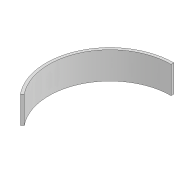
# Autodesk Inventor part: Ball_plate
Saved by Autodesk Inventor 2022 (Build 260153000, 153)
## iProperties
Created: 2022-08-08
Part Number: Ball_plate
Material: Generic
Document SubType Name: Modeling
Designer: dell
Density: 1 g/cm^3
Appearance: Default
Author: dell
Autodesk Inventor part; units mm, degrees
ref_plane "YZ Plane" through (0, 0, 0) normal (1, 0, 0) x (0, 1, 0)
ref_plane "XZ Plane" through (0, 0, 0) normal (0, 1, 0) x (-1, 0, 0)
ref_plane "XY Plane" through (0, 0, 0) normal (0, 0, 1) x (1, 0, 0)
sketch "Sketch2" plane through (0, 0, 0) normal (0, 1, 0) x (-1, 0, 0)
  arc A0 (0, 0) -> (35, 73.2843) centre (0, 45) ccw
  arc A1 (0, -2) -> (36.5556, 74.5413) centre (0, 45) ccw
  line L0 (0, 0) -> (0, -2)
  line L1 (36.5556, 74.5413) -> (35, 73.2843)
  dimension "d14" = 45
  dimension "d15" = 47
  dimension "d17" = 2
  dimension "d18" = 35
  constraints: 4 end point, 4 point on circle, 3 line through centre, 2 centre point, 1 vertical
  measures "d14" radius of A0
  measures "d15" radius of A1
  measures "d17" distance of L0.start L0.end
  measures "d18" horizontal distance of L0.start L1.end
extrude "Extrusion1" add sketch "Sketch2" along normal blind 20
body "Solid2"
